Autodesk Fusion 360 part; units mm, degrees
(part 12 of 25)
  arc A2406 (61.3719, 8.262) -> (61.2504, 7.9686) centre (61.3112, 8.1153) ccw
  arc A2407 (57.5323, 7.7343) -> (57.3078, 7.9588) centre (57.4201, 7.8465) ccw
  arc A2408 (58.1296, 7.9686) -> (58.0081, 8.262) centre (58.0689, 8.1153) ccw
  arc A2409 (54.9923, 7.7343) -> (54.7678, 7.9588) centre (54.8801, 7.8465) ccw
  arc A2410 (65.6889, 8.274) -> (65.6889, 7.9565) centre (65.6889, 8.1152) ccw
  line L833 (52.07, 7.5765) -> (51.8, 7.8465)
  line L834 (58.0689, 8.1153) -> (57.42, 7.8465)
  arc A2411 (56.9749, 34.0406) -> (57.2924, 34.0406) centre (57.1337, 34.0406) ccw
  arc A2412 (56.987, 34.4786) -> (57.2804, 34.6001) centre (57.1337, 34.5394) ccw
  arc A2413 (47.9089, 8.274) -> (47.9089, 7.9565) centre (47.9089, 8.1152) ccw
  line L835 (46.72, 7.8465) -> (46.6979, 7.8557)
  arc A2414 (55.2821, 35.2406) -> (55.0576, 35.4651) centre (55.1698, 35.3528) ccw
  line L836 (46.6979, 13.1749) -> (46.7828, 13.2598)
  line L837 (53.6911, 8.1153) -> (52.9889, 8.1153)
  arc A2415 (61.3111, 7.9565) -> (61.3111, 8.274) centre (61.3111, 8.1152) ccw
  line L838 (49.8, 7.8465) -> (49.53, 7.5765)
  arc A2416 (47.3723, 7.7343) -> (47.1478, 7.9588) centre (47.2601, 7.8465) ccw
  arc A2417 (46.8951, 13.1476) -> (46.6706, 13.3721) centre (46.7829, 13.2599) ccw
  arc A2418 (46.8566, 13.1749) -> (46.5391, 13.1749) centre (46.6979, 13.1749) ccw
  arc A2419 (46.5856, 13.2872) -> (46.8102, 13.0626) centre (46.6979, 13.1749) ccw
  arc A2420 (51.1511, 7.9565) -> (51.1511, 8.274) centre (51.1511, 8.1152) ccw
  line L839 (47.26, 7.8465) -> (46.99, 7.5765)
  arc A2421 (47.1993, 7.9932) -> (47.3208, 7.6999) centre (47.2601, 7.8466) ccw
  arc A2422 (48.6719, 8.262) -> (48.5504, 7.9686) centre (48.6112, 8.1153) ccw
  arc A2423 (49.1992, 7.6999) -> (49.3207, 7.9932) centre (49.26, 7.8466) ccw
  line L840 (49.26, 7.8465) -> (48.6111, 8.1153)
  line L841 (49.53, 7.5765) -> (49.26, 7.8465)
  line L842 (46.6979, 7.8557) -> (46.6979, 13.1749)
  line L843 (46.99, 7.5765) -> (46.72, 7.8465)
  line L844 (50.4489, 8.1153) -> (49.8, 7.8465)
  line L845 (48.6111, 8.1153) -> (47.9089, 8.1153)
  line L846 (57.1337, 34.0406) -> (57.1337, 34.5394)
  line L847 (56.88, 7.8465) -> (56.2311, 8.1153)
  arc A2424 (48.6111, 7.9565) -> (48.6111, 8.274) centre (48.6111, 8.1152) ccw
  arc A2425 (46.8322, 7.9588) -> (46.6077, 7.7343) centre (46.72, 7.8465) ccw
  line L848 (54.6263, 34.5394) -> (54.6263, 34.0406)
  arc A2426 (54.2792, 7.6999) -> (54.4007, 7.9932) centre (54.34, 7.8466) ccw
  arc A2427 (49.4177, 7.6888) -> (49.6423, 7.4643) centre (49.53, 7.5765) ccw
  arc A2428 (60.6696, 7.9686) -> (60.5481, 8.262) centre (60.6089, 8.1153) ccw
  arc A2429 (53.6911, 7.9565) -> (53.6911, 8.274) centre (53.6911, 8.1152) ccw
  arc A2430 (47.9696, 7.9686) -> (47.8481, 8.262) centre (47.9089, 8.1153) ccw
  arc A2431 (54.4796, 34.6001) -> (54.773, 34.4786) centre (54.6263, 34.5393) ccw
  arc A2432 (57.0895, 35.0609) -> (56.7962, 34.9394) centre (56.9429, 35.0001) ccw
  arc A2433 (54.785, 34.5394) -> (54.4676, 34.5394) centre (54.6263, 34.5394) ccw
  line L849 (59.69, 7.5765) -> (59.42, 7.8465)
  arc A2434 (54.4676, 34.0406) -> (54.785, 34.0406) centre (54.6263, 34.0406) ccw
  line L850 (54.8172, 35.0002) -> (54.6263, 34.5394)
  arc A2435 (49.4177, 7.4643) -> (49.6423, 7.6888) centre (49.53, 7.5765) ccw
  arc A2436 (46.8777, 7.6888) -> (47.1023, 7.4643) centre (46.99, 7.5766) ccw
  arc A2437 (54.9638, 34.9394) -> (54.6705, 35.0609) centre (54.8172, 35.0002) ccw
  arc A2438 (46.6592, 7.6999) -> (46.7807, 7.9932) centre (46.7199, 7.8465) ccw
  arc A2439 (50.5096, 7.9686) -> (50.3881, 8.262) centre (50.4489, 8.1153) ccw
  line L851 (61.3111, 8.1153) -> (60.6089, 8.1153)
  line L852 (55.1698, 35.3528) -> (54.8172, 35.0002)
  line L853 (47.9089, 8.1153) -> (47.26, 7.8465)
  arc A2440 (54.4977, 7.4643) -> (54.7223, 7.6888) centre (54.61, 7.5766) ccw
  arc A2441 (53.7519, 8.262) -> (53.6304, 7.9686) centre (53.6912, 8.1153) ccw
  line L854 (57.42, 7.8465) -> (57.15, 7.5765)
  arc A2442 (54.4522, 7.9588) -> (54.2277, 7.7343) centre (54.3399, 7.8466) ccw
  arc A2443 (57.2924, 34.5394) -> (56.9749, 34.5394) centre (57.1337, 34.5394) ccw
  line L855 (56.9428, 35.0002) -> (56.5902, 35.3528)
  line L856 (54.34, 7.8465) -> (53.6911, 8.1153)
  arc A2444 (49.9123, 7.7343) -> (49.6878, 7.9588) centre (49.8, 7.8466) ccw
  arc A2445 (55.6914, 35.397) -> (55.5699, 35.6904) centre (55.6307, 35.5437) ccw
  arc A2446 (49.7393, 7.9932) -> (49.8608, 7.6999) centre (49.8, 7.8466) ccw
  arc A2447 (55.1091, 35.4995) -> (55.2306, 35.2062) centre (55.1698, 35.3529) ccw
  arc A2448 (56.5294, 35.2062) -> (56.6509, 35.4995) centre (56.5902, 35.3529) ccw
  arc A2449 (54.7049, 35.1124) -> (54.9294, 34.8879) centre (54.8172, 35.0002) ccw
  line L857 (68.0202, 17.5728) -> (67.5594, 17.7637)
  arc A2450 (56.8306, 34.8879) -> (57.0551, 35.1124) centre (56.9429, 35.0001) ccw
  arc A2451 (68.7224, 16.7594) -> (68.4049, 16.7594) centre (68.5636, 16.7594) ccw
  arc A2452 (54.9043, 18.4353) -> (55.1976, 18.5568) centre (55.051, 18.496) ccw
  arc A2453 (49.3722, 7.9588) -> (49.1477, 7.7343) centre (49.26, 7.8465) ccw
  arc A2454 (46.6362, 13.3206) -> (46.9295, 13.1991) centre (46.7828, 13.2598) ccw
  line L858 (57.1337, 34.5394) -> (56.9428, 35.0002)
  arc A2455 (56.1901, 35.6904) -> (56.0686, 35.397) centre (56.1294, 35.5437) ccw
  arc A2456 (46.8777, 7.4643) -> (47.1023, 7.6888) centre (46.99, 7.5766) ccw
  arc A2457 (55.6306, 35.7024) -> (55.6306, 35.3849) centre (55.6306, 35.5436) ccw
  line L859 (67.5594, 15.2563) -> (68.0202, 15.4472)
  arc A2458 (67.0606, 17.9224) -> (67.0606, 17.6049) centre (67.0606, 17.7636) ccw
  line L860 (67.0606, 17.7637) -> (66.5998, 17.5728)
  arc A2459 (67.5594, 17.6049) -> (67.5594, 17.9224) centre (67.5594, 17.7636) ccw
  arc A2460 (55.1632, 18.6083) -> (54.9387, 18.3838) centre (55.051, 18.496) ccw
  arc A2461 (67.9079, 15.5594) -> (68.1324, 15.3349) centre (68.0202, 15.4472) ccw
  arc A2462 (67.1214, 17.617) -> (66.9999, 17.9104) centre (67.0606, 17.7637) ccw
  arc A2463 (66.7121, 17.4606) -> (66.4876, 17.6851) centre (66.5999, 17.5728) ccw
  arc A2464 (47.1204, 13.6599) -> (46.827, 13.7814) centre (46.9737, 13.7207) ccw
  line L861 (66.5998, 15.4472) -> (67.0606, 15.2563)
  line L862 (46.7828, 13.2598) -> (46.9737, 13.7206)
  arc A2465 (66.9999, 15.1096) -> (67.1214, 15.403) centre (67.0606, 15.2563) ccw
  line L863 (67.5594, 17.7637) -> (67.0606, 17.7637)
  arc A2466 (68.2262, 15.8606) -> (68.5195, 15.7391) centre (68.3728, 15.7999) ccw
  arc A2467 (54.7898, 33.3826) -> (55.0144, 33.6072) centre (54.9021, 33.4949) ccw
  arc A2468 (68.4851, 15.6876) -> (68.2606, 15.9121) centre (68.3728, 15.7999) ccw
  arc A2469 (57.7032, 16.0683) -> (57.4787, 15.8438) centre (57.591, 15.9561) ccw
  line L864 (66.5149, 17.4879) -> (58.8251, 17.4879)
  arc A2470 (54.9294, 33.6921) -> (54.7049, 33.4676) centre (54.8172, 33.5799) ccw
  line L865 (54.9021, 33.4949) -> (54.9021, 18.8555)
  arc A2471 (46.7586, 8.0024) -> (46.6372, 7.709) centre (46.6979, 7.8557) ccw
  arc A2472 (67.9594, 17.4262) -> (68.0809, 17.7195) centre (68.0202, 17.5728) ccw
  arc A2473 (67.6201, 17.9104) -> (67.4986, 17.617) centre (67.5593, 17.7637) ccw
  line L866 (54.9021, 18.8555) -> (55.051, 18.4961)
  line L867 (55.6306, 35.5437) -> (55.1698, 35.3528)
  line L868 (66.5998, 17.5728) -> (66.5149, 17.4879)
  arc A2474 (57.9268, 15.8276) -> (57.8053, 15.5343) centre (57.8661, 15.6809) ccw
  line L869 (66.5149, 15.5321) -> (66.5998, 15.4472)
  line L870 (56.5902, 35.3528) -> (56.1294, 35.5437)
  line L871 (68.5637, 16.2606) -> (68.5637, 16.7594)
  arc A2475 (54.773, 34.1014) -> (54.4796, 33.9799) centre (54.6263, 34.0406) ccw
  arc A2476 (67.4986, 15.403) -> (67.6201, 15.1096) centre (67.5593, 15.2563) ccw
  arc A2477 (46.5391, 7.8557) -> (46.8566, 7.8557) centre (46.6979, 7.8557) ccw
  arc A2478 (66.5391, 17.7195) -> (66.6606, 17.4262) centre (66.5999, 17.5729) ccw
  line L872 (54.6263, 34.0406) -> (54.8172, 33.5798)
  arc A2479 (68.5195, 17.2809) -> (68.2262, 17.1594) centre (68.3728, 17.2202) ccw
  arc A2480 (68.1324, 17.6851) -> (67.9079, 17.4606) centre (68.0202, 17.5728) ccw
  arc A2481 (54.6705, 33.5191) -> (54.9638, 33.6406) centre (54.8172, 33.5799) ccw
  arc A2482 (68.417, 16.6986) -> (68.7104, 16.8201) centre (68.5637, 16.7594) ccw
  arc A2483 (56.7024, 35.4651) -> (56.4779, 35.2406) centre (56.5902, 35.3529) ccw
  arc A2484 (68.2606, 17.1079) -> (68.4851, 17.3324) centre (68.3728, 17.2202) ccw
  arc A2485 (58.2255, 15.6909) -> (58.2255, 15.3734) centre (58.2255, 15.5321) ccw
  line L873 (56.1294, 35.5437) -> (55.6306, 35.5437)
  arc A2486 (66.4026, 17.6002) -> (66.6272, 17.3756) centre (66.5149, 17.4879) ccw
  arc A2487 (66.6272, 15.6444) -> (66.4026, 15.4198) centre (66.5149, 15.5321) ccw
  arc A2488 (56.1294, 35.3849) -> (56.1294, 35.7024) centre (56.1294, 35.5436) ccw
  line L874 (57.8661, 15.681) -> (58.2255, 15.5321)
  line L875 (68.3728, 17.2202) -> (68.0202, 17.5728)
  arc A2489 (68.5588, 2.0638) -> (68.5588, 1.7463) centre (68.5588, 1.9051) ccw
  arc A2490 (3.696, 3.0163) -> (3.696, 3.3338) centre (3.696, 3.1751) ccw
  arc A2491 (32.964, 1.7463) -> (32.964, 2.0638) centre (32.964, 1.9051) ccw
  line L876 (55.051, 18.4961) -> (57.591, 15.9561)
  arc A2492 (5.0673, 2.6987) -> (5.0673, 2.3813) centre (5.0673, 2.54) ccw
  arc A2493 (66.6606, 15.5938) -> (66.5391, 15.3005) centre (66.5999, 15.4472) ccw
  arc A2494 (57.4787, 15.8438) -> (57.7032, 16.0683) centre (57.591, 15.9561) ccw
  line L877 (68.5637, 16.7594) -> (68.3728, 17.2202)
  arc A2495 (57.7538, 15.5687) -> (57.9783, 15.7932) centre (57.8661, 15.681) ccw
  arc A2496 (73.5277, 1.1113) -> (73.5277, 1.4287) centre (73.5277, 1.27) ccw
  arc A2497 (54.7434, 18.8555) -> (55.0609, 18.8555) centre (54.9021, 18.8555) ccw
  arc A2498 (55.0488, 18.9162) -> (54.7554, 18.7947) centre (54.9021, 18.8555) ccw
  arc A2499 (68.7104, 16.1999) -> (68.417, 16.3214) centre (68.5637, 16.2607) ccw
  arc A2500 (72.4814, 2.3813) -> (72.4814, 2.6987) centre (72.4814, 2.54) ccw
  line L878 (54.8172, 33.5798) -> (54.9021, 33.4949)
  line L879 (58.2255, 15.5321) -> (66.5149, 15.5321)
  arc A2501 (66.5149, 15.3734) -> (66.5149, 15.6909) centre (66.5149, 15.5321) ccw
  arc A2502 (58.8251, 17.6466) -> (58.8251, 17.3291) centre (58.8251, 17.4879) ccw
  arc A2503 (67.5594, 15.0976) -> (67.5594, 15.4151) centre (67.5594, 15.2564) ccw
  line L880 (56.8579, 19.4551) -> (56.8579, 33.4949)
  arc A2504 (5.0673, 2.3813) -> (5.0673, 2.6987) centre (5.0673, 2.54) ccw
  arc A2505 (68.5588, 2.6987) -> (68.5588, 2.3813) centre (68.5588, 2.54) ccw
  arc A2506 (4.331, 2.3813) -> (4.331, 2.6987) centre (4.331, 2.54) ccw
  arc A2507 (6.4386, 3.3338) -> (6.4386, 3.0163) centre (6.4386, 3.1751) ccw
  line L881 (67.0606, 15.2563) -> (67.5594, 15.2563)
  arc A2508 (67.0606, 15.4151) -> (67.0606, 15.0976) centre (67.0606, 15.2564) ccw
  arc A2509 (68.0809, 15.3005) -> (67.9594, 15.5938) centre (68.0202, 15.4472) ccw
  arc A2510 (84.2253, 2.3813) -> (84.2253, 2.6987) centre (84.2253, 2.54) ccw
  arc A2511 (66.4876, 15.3349) -> (66.7121, 15.5594) centre (66.5999, 15.4472) ccw
  arc A2512 (82.5144, 2.6987) -> (82.5144, 2.3813) centre (82.5144, 2.54) ccw
  arc A2513 (0.7747, 3.3338) -> (0.7747, 3.0163) centre (0.7747, 3.1751) ccw
  arc A2514 (58.1647, 15.3854) -> (58.2862, 15.6788) centre (58.2255, 15.5321) ccw
  arc A2515 (55.0609, 33.4949) -> (54.7434, 33.4949) centre (54.9021, 33.4949) ccw
  arc A2516 (12.6114, 3.0163) -> (12.6114, 3.3338) centre (12.6114, 3.1751) ccw
  arc A2517 (13.97, 3.3338) -> (13.97, 3.0163) centre (13.97, 3.1751) ccw
  arc A2518 (56.7456, 33.6072) -> (56.9702, 33.3826) centre (56.8579, 33.4949) ccw
  arc A2519 (68.4049, 16.2606) -> (68.7224, 16.2606) centre (68.5636, 16.2606) ccw
  arc A2520 (56.6991, 19.4551) -> (57.0166, 19.4551) centre (56.8578, 19.4551) ccw
  line L882 (56.9428, 33.5798) -> (57.1337, 34.0406)
  arc A2521 (57.2804, 33.9799) -> (56.987, 34.1014) centre (57.1337, 34.0406) ccw
  arc A2522 (5.0673, 3.3338) -> (5.0673, 3.0163) centre (5.0673, 3.1751) ccw
  arc A2523 (13.97, 3.0163) -> (13.97, 3.3338) centre (13.97, 3.1751) ccw
  line L883 (57.591, 15.9561) -> (57.8661, 15.681)
  arc A2524 (57.0551, 33.4676) -> (56.8306, 33.6921) centre (56.9429, 33.5799) ccw
  line L884 (68.0202, 15.4472) -> (68.3728, 15.7998)
  line L885 (68.3728, 15.7998) -> (68.5637, 16.2606)
  arc A2525 (5.0673, 3.0163) -> (5.0673, 3.3338) centre (5.0673, 3.1751) ccw
  arc A2526 (74.9658, 1.4287) -> (74.9658, 1.1113) centre (74.9658, 1.27) ccw
  arc A2527 (58.7128, 17.3756) -> (58.9373, 17.6002) centre (58.8251, 17.4879) ccw
  line L886 (56.8579, 33.4949) -> (56.9428, 33.5798)
  arc A2528 (40.64, 4.9212) -> (40.64, 5.2388) centre (40.64, 5.08) ccw
  arc A2529 (84.2253, 1.1113) -> (84.2253, 1.4287) centre (84.2253, 1.27) ccw
  arc A2530 (6.4132, 4.6038) -> (6.4132, 4.2862) centre (6.4132, 4.445) ccw
  arc A2531 (81.4682, 1.4287) -> (81.4682, 1.1113) centre (81.4682, 1.27) ccw
  arc A2532 (14.6936, 2.6987) -> (14.6936, 2.3813) centre (14.6936, 2.54) ccw
  arc A2533 (0.7747, 1.4287) -> (0.7747, 1.1113) centre (0.7747, 1.27) ccw
  arc A2534 (0.7747, 2.6987) -> (0.7747, 2.3813) centre (0.7747, 2.54) ccw
  arc A2535 (0.7747, 2.0638) -> (0.7747, 1.7463) centre (0.7747, 1.9051) ccw
  line L887 (58.8251, 17.4879) -> (56.8579, 19.4551)
  arc A2536 (68.5588, 1.4287) -> (68.5588, 1.1113) centre (68.5588, 1.27) ccw
  arc A2537 (33.1022, 3.6513) -> (33.1022, 3.9688) centre (33.1022, 3.81) ccw
  arc A2538 (13.97, 3.9688) -> (13.97, 3.6513) centre (13.97, 3.81) ccw
  arc A2539 (13.2464, 2.3813) -> (13.2464, 2.6987) centre (13.2464, 2.54) ccw
  arc A2540 (82.2548, 2.0638) -> (82.2548, 1.7463) centre (82.2548, 1.9051) ccw
  arc A2541 (41.4632, 5.2388) -> (41.4632, 4.9212) centre (41.4632, 5.08) ccw
  arc A2542 (15.3286, 3.3338) -> (15.3286, 3.0163) centre (15.3286, 3.1751) ccw
  arc A2543 (72.4814, 3.0163) -> (72.4814, 3.3338) centre (72.4814, 3.1751) ccw
  arc A2544 (66.5149, 17.3291) -> (66.5149, 17.6466) centre (66.5149, 17.4879) ccw
  arc A2545 (72.72, 3.6513) -> (72.72, 3.9688) centre (72.72, 3.81) ccw
  arc A2546 (13.97, 2.3813) -> (13.97, 2.6987) centre (13.97, 2.54) ccw
  arc A2547 (73.405, 4.2862) -> (73.405, 4.6038) centre (73.405, 4.445) ccw
  arc A2548 (40.64, 5.2388) -> (40.64, 4.9212) centre (40.64, 5.08) ccw
  arc A2549 (38.1, 5.2388) -> (38.1, 4.9212) centre (38.1, 5.08) ccw
  arc A2550 (41.9535, 4.9212) -> (41.9535, 5.2388) centre (41.9535, 5.08) ccw
  arc A2551 (3.9718, 4.9212) -> (3.9718, 5.2388) centre (3.9718, 5.08) ccw
  arc A2552 (34.3335, 4.9212) -> (34.3335, 5.2388) centre (34.3335, 5.08) ccw
  arc A2553 (31.7935, 4.9212) -> (31.7935, 5.2388) centre (31.7935, 5.08) ccw
  arc A2554 (39.8168, 4.9212) -> (39.8168, 5.2388) centre (39.8168, 5.08) ccw
  arc A2555 (82.5144, 3.3338) -> (82.5144, 3.0163) centre (82.5144, 3.1751) ccw
  line L888 (34.2465, 5.08) -> (34.3335, 5.08)
  line L889 (41.4632, 5.08) -> (41.9535, 5.08)
  arc A2556 (84.2253, 1.7463) -> (84.2253, 2.0638) centre (84.2253, 1.9051) ccw
  arc A2557 (5.8036, 2.6987) -> (5.8036, 2.3813) centre (5.8036, 2.54) ccw
  arc A2558 (15.0528, 5.2388) -> (15.0528, 4.9212) centre (15.0528, 5.08) ccw
  arc A2559 (80.0301, 1.1113) -> (80.0301, 1.4287) centre (80.0301, 1.27) ccw
  arc A2560 (13.97, 3.6513) -> (13.97, 3.9688) centre (13.97, 3.81) ccw
  arc A2561 (84.2253, 3.6513) -> (84.2253, 3.9688) centre (84.2253, 3.81) ccw
  arc A2562 (6.477, 3.9688) -> (6.477, 3.6513) centre (6.477, 3.81) ccw
  arc A2563 (12.8872, 4.9212) -> (12.8872, 5.2388) centre (12.8872, 5.08) ccw
  arc A2564 (13.97, 2.6987) -> (13.97, 2.3813) centre (13.97, 2.54) ccw
  arc A2565 (37.2768, 4.9212) -> (37.2768, 5.2388) centre (37.2768, 5.08) ccw
  arc A2566 (72.7411, 1.7463) -> (72.7411, 2.0638) centre (72.7411, 1.9051) ccw
  arc A2567 (32.964, 1.1113) -> (32.964, 1.4287) centre (32.964, 1.27) ccw
  arc A2568 (68.4207, 3.9688) -> (68.4207, 3.6513) centre (68.4207, 3.81) ccw
  arc A2569 (57.0166, 33.4949) -> (56.6991, 33.4949) centre (56.8578, 33.4949) ccw
  arc A2570 (84.2253, 3.0163) -> (84.2253, 3.3338) centre (84.2253, 3.1751) ccw
  arc A2571 (56.9702, 19.5673) -> (56.7456, 19.3428) centre (56.8579, 19.455) ccw
  arc A2572 (32.964, 2.3813) -> (32.964, 2.6987) centre (32.964, 2.54) ccw
  arc A2573 (56.7962, 33.6406) -> (57.0895, 33.5191) centre (56.9428, 33.5799) ccw
  arc A2574 (40.64, 5.8738) -> (40.64, 5.5562) centre (40.64, 5.715) ccw
  arc A2575 (62.1865, 5.2388) -> (62.1865, 4.9212) centre (62.1865, 5.08) ccw
  line L890 (54.5665, 5.08) -> (54.6535, 5.08)
  arc A2576 (3.4036, 6.1913) -> (3.4036, 6.5088) centre (3.4036, 6.3501) ccw
  arc A2577 (0.7747, 4.6038) -> (0.7747, 4.2862) centre (0.7747, 4.445) ccw
  arc A2578 (6.731, 6.5088) -> (6.731, 6.1913) centre (6.731, 6.3501) ccw
  arc A2579 (68.5588, 3.3338) -> (68.5588, 3.0163) centre (68.5588, 3.1751) ccw
  arc A2580 (82.2759, 3.9688) -> (82.2759, 3.6513) centre (82.2759, 3.81) ccw
  arc A2581 (52.0265, 5.2388) -> (52.0265, 4.9212) centre (52.0265, 5.08) ccw
  arc A2582 (38.9232, 5.2388) -> (38.9232, 4.9212) centre (38.9232, 5.08) ccw
  arc A2583 (62.2735, 4.9212) -> (62.2735, 5.2388) centre (62.2735, 5.08) ccw
  line L891 (59.6465, 5.08) -> (59.7335, 5.08)
  line L892 (46.9465, 5.08) -> (47.0335, 5.08)
  arc A2584 (84.2253, 4.9212) -> (84.2253, 5.2388) centre (84.2253, 5.08) ccw
  arc A2585 (36.7865, 5.2388) -> (36.7865, 4.9212) centre (36.7865, 5.08) ccw
  line L893 (38.9232, 5.08) -> (39.8168, 5.08)
  line L894 (64.7265, 5.08) -> (64.8135, 5.08)
  line L895 (67.2665, 5.08) -> (67.3535, 5.08)
  arc A2586 (15.6337, 5.8738) -> (15.6337, 5.5562) centre (15.6337, 5.715) ccw
  arc A2587 (40.64, 5.5562) -> (40.64, 5.8738) centre (40.64, 5.715) ccw
  arc A2588 (74.7818, 5.8738) -> (74.7818, 5.5562) centre (74.7818, 5.715) ccw
  arc A2589 (3.4036, 5.5562) -> (3.4036, 5.8738) centre (3.4036, 5.715) ccw
  arc A2590 (67.3535, 4.9212) -> (67.3535, 5.2388) centre (67.3535, 5.08) ccw
  arc A2591 (52.1135, 4.9212) -> (52.1135, 5.2388) centre (52.1135, 5.08) ccw
  arc A2592 (54.6535, 4.9212) -> (54.6535, 5.2388) centre (54.6535, 5.08) ccw
  arc A2593 (12.6114, 4.2862) -> (12.6114, 4.6038) centre (12.6114, 4.445) ccw
  arc A2594 (15.3286, 4.6038) -> (15.3286, 4.2862) centre (15.3286, 4.445) ccw
  arc A2595 (38.1, 4.9212) -> (38.1, 5.2388) centre (38.1, 5.08) ccw
  arc A2596 (64.7265, 5.2388) -> (64.7265, 4.9212) centre (64.7265, 5.08) ccw
  arc A2597 (32.964, 3.0163) -> (32.964, 3.3338) centre (32.964, 3.1751) ccw
  arc A2598 (0.7747, 5.2388) -> (0.7747, 4.9212) centre (0.7747, 5.08) ccw
  arc A2599 (79.9074, 4.2862) -> (79.9074, 4.6038) centre (79.9074, 4.445) ccw
  arc A2600 (44.4065, 5.2388) -> (44.4065, 4.9212) centre (44.4065, 5.08) ccw
  arc A2601 (57.1065, 5.2388) -> (57.1065, 4.9212) centre (57.1065, 5.08) ccw
  arc A2602 (12.3063, 5.5562) -> (12.3063, 5.8738) centre (12.3063, 5.715) ccw
  arc A2603 (3.7214, 4.2862) -> (3.7214, 4.6038) centre (3.7214, 4.445) ccw
  arc A2604 (64.8135, 4.9212) -> (64.8135, 5.2388) centre (64.8135, 5.08) ccw
  arc A2605 (84.2253, 5.5562) -> (84.2253, 5.8738) centre (84.2253, 5.715) ccw
  arc A2606 (34.2465, 5.2388) -> (34.2465, 4.9212) centre (34.2465, 5.08) ccw
  arc A2607 (44.4935, 4.9212) -> (44.4935, 5.2388) centre (44.4935, 5.08) ccw
  line L896 (36.7865, 5.08) -> (37.2768, 5.08)
  arc A2608 (73.7116, 5.5562) -> (73.7116, 5.8738) centre (73.7116, 5.715) ccw
  arc A2609 (84.2253, 4.2862) -> (84.2253, 4.6038) centre (84.2253, 4.445) ccw
  arc A2610 (0.7747, 3.9688) -> (0.7747, 3.6513) centre (0.7747, 3.81) ccw
  arc A2611 (3.6576, 3.6513) -> (3.6576, 3.9688) centre (3.6576, 3.81) ccw
  arc A2612 (49.4865, 5.2388) -> (49.4865, 4.9212) centre (49.4865, 5.08) ccw
  arc A2613 (75.0884, 4.6038) -> (75.0884, 4.2862) centre (75.0884, 4.445) ccw
  arc A2614 (59.7335, 4.9212) -> (59.7335, 5.2388) centre (59.7335, 5.08) ccw
  arc A2615 (69.8065, 5.2388) -> (69.8065, 4.9212) centre (69.8065, 5.08) ccw
  arc A2616 (6.1628, 5.2388) -> (6.1628, 4.9212) centre (6.1628, 5.08) ccw
  arc A2617 (81.5908, 4.6038) -> (81.5908, 4.2862) centre (81.5908, 4.445) ccw
  arc A2618 (29.4986, 5.5562) -> (29.4986, 5.8738) centre (29.4986, 5.715) ccw
  arc A2619 (38.1, 5.8738) -> (38.1, 5.5562) centre (38.1, 5.715) ccw
  arc A2620 (44.4935, 7.4612) -> (44.4935, 7.7788) centre (44.4935, 7.62) ccw
  arc A2621 (40.64, 6.8262) -> (40.64, 7.1438) centre (40.64, 6.985) ccw
  arc A2622 (82.1916, 6.5088) -> (82.1916, 6.1913) centre (82.1916, 6.3501) ccw
  arc A2623 (57.1935, 4.9212) -> (57.1935, 5.2388) centre (57.1935, 5.08) ccw
  arc A2624 (80.214, 5.5562) -> (80.214, 5.8738) centre (80.214, 5.715) ccw
  arc A2625 (31.7935, 7.4612) -> (31.7935, 7.7788) centre (31.7935, 7.62) ccw
  arc A2626 (34.2465, 7.7788) -> (34.2465, 7.4612) centre (34.2465, 7.62) ccw
  arc A2627 (46.9465, 5.2388) -> (46.9465, 4.9212) centre (46.9465, 5.08) ccw
  arc A2628 (41.4632, 7.7788) -> (41.4632, 7.4612) centre (41.4632, 7.62) ccw
  arc A2629 (54.5665, 5.2388) -> (54.5665, 4.9212) centre (54.5665, 5.08) ccw
  arc A2630 (3.9972, 7.4612) -> (3.9972, 7.7788) centre (3.9972, 7.62) ccw
  arc A2631 (40.64, 7.1438) -> (40.64, 6.8262) centre (40.64, 6.985) ccw
  arc A2632 (12.3063, 6.1913) -> (12.3063, 6.5088) centre (12.3063, 6.3501) ccw
  arc A2633 (15.6337, 6.5088) -> (15.6337, 6.1913) centre (15.6337, 6.3501) ccw
  arc A2634 (49.5735, 4.9212) -> (49.5735, 5.2388) centre (49.5735, 5.08) ccw
  arc A2635 (70.7429, 6.8262) -> (70.7429, 7.1438) centre (70.7429, 6.985) ccw
  arc A2636 (0.7747, 7.7788) -> (0.7747, 7.4612) centre (0.7747, 7.62) ccw
  line L897 (57.1065, 5.08) -> (57.1935, 5.08)
  line L898 (62.1865, 5.08) -> (62.2735, 5.08)
  arc A2637 (0.7747, 6.5088) -> (0.7747, 6.1913) centre (0.7747, 6.3501) ccw
  arc A2638 (67.2665, 5.2388) -> (67.2665, 4.9212) centre (67.2665, 5.08) ccw
  arc A2639 (38.1, 7.7788) -> (38.1, 7.4612) centre (38.1, 7.62) ccw
  arc A2640 (70.2277, 7.1438) -> (70.2277, 6.8262) centre (70.2277, 6.985) ccw
  arc A2641 (34.3335, 7.4612) -> (34.3335, 7.7788) centre (34.3335, 7.62) ccw
  arc A2642 (79.3067, 6.1913) -> (79.3067, 6.5088) centre (79.3067, 6.3501) ccw
  line L899 (38.1, 6.35) -> (40.64, 6.35)
  arc A2643 (15.6337, 7.1438) -> (15.6337, 6.8262) centre (15.6337, 6.985) ccw
  arc A2644 (38.1, 5.5562) -> (38.1, 5.8738) centre (38.1, 5.715) ccw
  arc A2645 (0.7747, 5.8738) -> (0.7747, 5.5562) centre (0.7747, 5.715) ccw
  arc A2646 (59.6465, 5.2388) -> (59.6465, 4.9212) centre (59.6465, 5.08) ccw
  arc A2647 (75.6891, 6.5088) -> (75.6891, 6.1913) centre (75.6891, 6.3501) ccw
  arc A2648 (40.64, 7.7788) -> (40.64, 7.4612) centre (40.64, 7.62) ccw
  arc A2649 (6.731, 5.8738) -> (6.731, 5.5562) centre (6.731, 5.715) ccw
  line L900 (46.9465, 7.62) -> (47.0335, 7.62)
  arc A2650 (40.64, 6.1913) -> (40.64, 6.5088) centre (40.64, 6.3501) ccw
  arc A2651 (47.0335, 7.4612) -> (47.0335, 7.7788) centre (47.0335, 7.62) ccw
  arc A2652 (6.1374, 7.7788) -> (6.1374, 7.4612) centre (6.1374, 7.62) ccw
  arc A2653 (3.4036, 6.8262) -> (3.4036, 7.1438) centre (3.4036, 6.985) ccw
  arc A2654 (38.1, 6.8262) -> (38.1, 7.1438) centre (38.1, 6.985) ccw
  arc A2655 (0.7747, 7.1438) -> (0.7747, 6.8262) centre (0.7747, 6.985) ccw
  arc A2656 (11.317, 7.4612) -> (11.317, 7.7788) centre (11.317, 7.62) ccw
  arc A2657 (81.2842, 5.8738) -> (81.2842, 5.5562) centre (81.2842, 5.715) ccw
  arc A2658 (28.8636, 6.1913) -> (28.8636, 6.5088) centre (28.8636, 6.3501) ccw
  arc A2659 (70.2277, 5.8738) -> (70.2277, 5.5562) centre (70.2277, 5.715) ccw
  line L901 (44.4065, 5.08) -> (44.4935, 5.08)
  arc A2660 (38.1, 7.1438) -> (38.1, 6.8262) centre (38.1, 6.985) ccw
  arc A2661 (41.9535, 7.4612) -> (41.9535, 7.7788) centre (41.9535, 7.62) ccw
  line L902 (49.4865, 5.08) -> (49.5735, 5.08)
  arc A2662 (47.0335, 4.9212) -> (47.0335, 5.2388) centre (47.0335, 5.08) ccw
  line L903 (52.0265, 5.08) -> (52.1135, 5.08)
  arc A2663 (11.952, 6.8262) -> (11.952, 7.1438) centre (11.952, 6.985) ccw
  arc A2664 (59.6465, 7.7788) -> (59.6465, 7.4612) centre (59.6465, 7.62) ccw
  arc A2665 (84.2253, 8.0963) -> (84.2253, 8.4138) centre (84.2253, 8.2551) ccw
  arc A2666 (54.6535, 7.4612) -> (54.6535, 7.7788) centre (54.6535, 7.62) ccw
  arc A2667 (40.64, 7.4612) -> (40.64, 7.7788) centre (40.64, 7.62) ccw
  line L904 (49.4865, 7.62) -> (49.5735, 7.62)
  line L905 (62.1865, 7.62) -> (62.2735, 7.62)
  arc A2668 (26.3236, 8.7313) -> (26.3236, 9.0488) centre (26.3236, 8.89) ccw
  arc A2669 (82.983, 8.4138) -> (82.983, 8.0963) centre (82.983, 8.2551) ccw
  arc A2670 (37.2768, 7.4612) -> (37.2768, 7.7788) centre (37.2768, 7.62) ccw
  line L906 (34.2465, 7.62) -> (34.3335, 7.62)
  arc A2671 (44.4065, 7.7788) -> (44.4065, 7.4612) centre (44.4065, 7.62) ccw
  arc A2672 (30.8264, 7.7788) -> (30.8264, 7.4612) centre (30.8264, 7.62) ccw
  arc A2673 (84.2253, 6.8262) -> (84.2253, 7.1438) centre (84.2253, 6.985) ccw
  arc A2674 (72.8043, 6.1913) -> (72.8043, 6.5088) centre (72.8043, 6.3501) ccw
  arc A2675 (54.5665, 7.7788) -> (54.5665, 7.4612) centre (54.5665, 7.62) ccw
  arc A2676 (15.0528, 7.7788) -> (15.0528, 7.4612) centre (15.0528, 7.62) ccw
  arc A2677 (27.5936, 7.4612) -> (27.5936, 7.7788) centre (27.5936, 7.62) ccw
  arc A2678 (44.7421, 8.0963) -> (44.7421, 8.4138) centre (44.7421, 8.2551) ccw
  arc A2679 (38.1, 7.4612) -> (38.1, 7.7788) centre (38.1, 7.62) ccw
  arc A2680 (39.8168, 7.4612) -> (39.8168, 7.7788) centre (39.8168, 7.62) ccw
  arc A2681 (52.1135, 7.4612) -> (52.1135, 7.7788) centre (52.1135, 7.62) ccw
  line L907 (69.8065, 7.62) -> (70.1079, 7.62)
  arc A2682 (26.9586, 8.0963) -> (26.9586, 8.4138) centre (26.9586, 8.2551) ccw
  arc A2683 (28.2286, 6.8262) -> (28.2286, 7.1438) centre (28.2286, 6.985) ccw
  arc A2684 (84.2253, 6.1913) -> (84.2253, 6.5088) centre (84.2253, 6.3501) ccw
  arc A2685 (82.4863, 7.1438) -> (82.4863, 6.8262) centre (82.4863, 6.985) ccw
  arc A2686 (13.448, 8.4138) -> (13.448, 8.0963) centre (13.448, 8.2551) ccw
  arc A2687 (70.3453, 6.5088) -> (70.3453, 6.1913) centre (70.3453, 6.3501) ccw
  arc A2688 (46.9465, 7.7788) -> (46.9465, 7.4612) centre (46.9465, 7.62) ccw
  arc A2689 (29.5564, 9.0488) -> (29.5564, 8.7313) centre (29.5564, 8.89) ccw
  arc A2690 (46.6979, 8.4138) -> (46.6979, 8.0963) centre (46.6979, 8.2551) ccw
  arc A2691 (38.1, 6.5088) -> (38.1, 6.1913) centre (38.1, 6.3501) ccw
  arc A2692 (52.0265, 7.7788) -> (52.0265, 7.4612) centre (52.0265, 7.62) ccw
  line L908 (57.1065, 7.62) -> (57.1935, 7.62)
  arc A2693 (59.7335, 7.4612) -> (59.7335, 7.7788) centre (59.7335, 7.62) ccw
  line L909 (64.7265, 7.62) -> (64.8135, 7.62)
  arc A2694 (38.9232, 7.7788) -> (38.9232, 7.4612) centre (38.9232, 7.62) ccw
  arc A2695 (67.2665, 7.7788) -> (67.2665, 7.4612) centre (67.2665, 7.62) ccw
  arc A2696 (69.4729, 8.0963) -> (69.4729, 8.4138) centre (69.4729, 8.2551) ccw
  arc A2697 (36.7865, 7.7788) -> (36.7865, 7.4612) centre (36.7865, 7.62) ccw
  arc A2698 (46.6979, 9.0488) -> (46.6979, 8.7313) centre (46.6979, 8.89) ccw
  arc A2699 (6.731, 7.1438) -> (6.731, 6.8262) centre (6.731, 6.985) ccw
  arc A2700 (68.8379, 8.7313) -> (68.8379, 9.0488) centre (68.8379, 8.89) ccw
  arc A2701 (82.5144, 7.7788) -> (82.5144, 7.4612) centre (82.5144, 7.62) ccw
  arc A2702 (64.8135, 7.4612) -> (64.8135, 7.7788) centre (64.8135, 7.62) ccw
  line L910 (59.6465, 7.62) -> (59.7335, 7.62)
  arc A2703 (4.1275, 8.7313) -> (4.1275, 9.0488) centre (4.1275, 8.89) ccw
  line L911 (52.0265, 7.62) -> (52.1135, 7.62)
  arc A2704 (84.2253, 8.7313) -> (84.2253, 9.0488) centre (84.2253, 8.89) ccw
  arc A2705 (0.7747, 10.3187) -> (0.7747, 10.0013) centre (0.7747, 10.16) ccw
  arc A2706 (30.1914, 8.4138) -> (30.1914, 8.0963) centre (30.1914, 8.2551) ccw
  arc A2707 (28.2864, 10.3187) -> (28.2864, 10.0013) centre (28.2864, 10.16) ccw
  arc A2708 (10.4521, 8.7313) -> (10.4521, 9.0488) centre (10.4521, 8.89) ccw
  arc A2709 (67.3535, 7.4612) -> (67.3535, 7.7788) centre (67.3535, 7.62) ccw
  line L912 (54.5665, 7.62) -> (54.6535, 7.62)
  arc A2710 (64.7265, 7.7788) -> (64.7265, 7.4612) centre (64.7265, 7.62) ccw
  arc A2711 (79.7385, 8.7313) -> (79.7385, 9.0488) centre (79.7385, 8.89) ccw
  arc A2712 (57.1065, 7.7788) -> (57.1065, 7.4612) centre (57.1065, 7.62) ccw
  arc A2713 (3.6263, 10.6363) -> (3.6263, 10.9537) centre (3.6263, 10.795) ccw
  arc A2714 (14.4213, 10.0013) -> (14.4213, 10.3187) centre (14.4213, 10.16) ccw
  arc A2715 (12.813, 9.0488) -> (12.813, 8.7313) centre (12.813, 8.89) ccw
  arc A2716 (12.4079, 10.3187) -> (12.4079, 10.0013) centre (12.4079, 10.16) ccw
  arc A2717 (81.6991, 10.0013) -> (81.6991, 10.3187) centre (81.6991, 10.16) ccw
  arc A2718 (6.0833, 9.6837) -> (6.0833, 9.3663) centre (6.0833, 9.525) ccw
  arc A2719 (84.2253, 7.4612) -> (84.2253, 7.7788) centre (84.2253, 7.62) ccw
  arc A2720 (62.1865, 7.7788) -> (62.1865, 7.4612) centre (62.1865, 7.62) ccw
  arc A2721 (69.8065, 7.7788) -> (69.8065, 7.4612) centre (69.8065, 7.62) ccw
  arc A2722 (46.6979, 10.3187) -> (46.6979, 10.0013) centre (46.6979, 10.16) ccw
  arc A2723 (66.0563, 10.0013) -> (66.0563, 10.3187) centre (66.0563, 10.16) ccw
  arc A2724 (76.313, 10.3187) -> (76.313, 10.0013) centre (76.313, 10.16) ccw
  arc A2725 (6.0833, 9.0488) -> (6.0833, 8.7313) centre (6.0833, 8.89) ccw
  arc A2726 (84.2253, 10.0013) -> (84.2253, 10.3187) centre (84.2253, 10.16) ccw
  arc A2727 (70.372, 10.0013) -> (70.372, 10.3187) centre (70.372, 10.16) ccw
  arc A2728 (83.6549, 10.3187) -> (83.6549, 10.0013) centre (83.6549, 10.16) ccw
  arc A2729 (49.4865, 7.7788) -> (49.4865, 7.4612) centre (49.4865, 7.62) ccw
  arc A2730 (4.1275, 10.0013) -> (4.1275, 10.3187) centre (4.1275, 10.16) ccw
  arc A2731 (83.5524, 9.0488) -> (83.5524, 8.7313) centre (83.5524, 8.89) ccw
  arc A2732 (6.0833, 8.4138) -> (6.0833, 8.0963) centre (6.0833, 8.2551) ccw
  arc A2733 (71.007, 9.3663) -> (71.007, 9.6837) centre (71.007, 9.525) ccw
  arc A2734 (57.1935, 7.4612) -> (57.1935, 7.7788) centre (57.1935, 7.62) ccw
  arc A2735 (0.7747, 10.9537) -> (0.7747, 10.6363) centre (0.7747, 10.795) ccw
  arc A2736 (10.682, 8.0963) -> (10.682, 8.4138) centre (10.682, 8.2551) ccw
  arc A2737 (25.0536, 10.0013) -> (25.0536, 10.3187) centre (25.0536, 10.16) ccw
  arc A2738 (28.9214, 9.6837) -> (28.9214, 9.3663) centre (28.9214, 9.525) ccw
  arc A2739 (0.7747, 8.4138) -> (0.7747, 8.0963) centre (0.7747, 8.2551) ccw
  arc A2740 (44.7421, 8.7313) -> (44.7421, 9.0488) centre (44.7421, 8.89) ccw
  line L913 (67.2665, 7.62) -> (67.3535, 7.62)
  arc A2741 (4.1275, 8.0963) -> (4.1275, 8.4138) centre (4.1275, 8.2551) ccw
  arc A2742 (16.1095, 10.3187) -> (16.1095, 10.0013) centre (16.1095, 10.16) ccw
  arc A2743 (83.6549, 9.6837) -> (83.6549, 9.3663) centre (83.6549, 9.525) ccw
  arc A2744 (62.2735, 7.4612) -> (62.2735, 7.7788) centre (62.2735, 7.62) ccw
  arc A2745 (71.6038, 9.0488) -> (71.6038, 8.7313) centre (71.6038, 8.89) ccw
  arc A2746 (70.1079, 7.4612) -> (70.1079, 7.7788) centre (70.1079, 7.62) ccw
  arc A2747 (0.7747, 9.0488) -> (0.7747, 8.7313) centre (0.7747, 8.89) ccw
  arc A2748 (49.5735, 7.4612) -> (49.5735, 7.7788) centre (49.5735, 7.62) ccw
  arc A2749 (70.3338, 10.3187) -> (70.3338, 10.0013) centre (70.3338, 10.16) ccw
  arc A2750 (25.6886, 9.3663) -> (25.6886, 9.6837) centre (25.6886, 9.525) ccw
  line L914 (70.3338, 10.16) -> (70.372, 10.16)
  line L915 (70.9688, 9.525) -> (71.007, 9.525)
  arc A2751 (12.4079, 9.6837) -> (12.4079, 9.3663) centre (12.4079, 9.525) ccw
  arc A2752 (84.2253, 9.3663) -> (84.2253, 9.6837) centre (84.2253, 9.525) ccw
  arc A2753 (81.4871, 9.3663) -> (81.4871, 9.6837) centre (81.4871, 9.525) ccw
  arc A2754 (69.102, 11.2713) -> (69.102, 11.5887) centre (69.102, 11.43) ccw
  arc A2755 (81.5916, 11.2713) -> (81.5916, 11.5887) centre (81.5916, 11.43) ccw
  arc A2756 (13.7795, 11.2713) -> (13.7795, 11.5887) centre (13.7795, 11.43) ccw
  arc A2757 (6.0833, 10.3187) -> (6.0833, 10.0013) centre (6.0833, 10.16) ccw
  arc A2758 (0.7747, 9.6837) -> (0.7747, 9.3663) centre (0.7747, 9.525) ccw
  arc A2759 (0.7747, 11.5887) -> (0.7747, 11.2713) centre (0.7747, 11.43) ccw
  arc A2760 (44.7421, 10.6363) -> (44.7421, 10.9537) centre (44.7421, 10.795) ccw
  arc A2761 (77.583, 11.5887) -> (77.583, 11.2713) centre (77.583, 11.43) ccw
  arc A2762 (66.216, 9.3663) -> (66.216, 9.6837) centre (66.216, 9.525) ccw
  arc A2763 (70.9688, 9.6837) -> (70.9688, 9.3663) centre (70.9688, 9.525) ccw
  arc A2764 (16.8945, 11.5887) -> (16.8945, 11.2713) centre (16.8945, 11.43) ccw
  arc A2765 (27.0164, 11.5887) -> (27.0164, 11.2713) centre (27.0164, 11.43) ccw
  arc A2766 (84.2253, 11.2713) -> (84.2253, 11.5887) centre (84.2253, 11.43) ccw
  arc A2767 (44.7421, 10.0013) -> (44.7421, 10.3187) centre (44.7421, 10.16) ccw
  arc A2768 (10.4521, 10.0013) -> (10.4521, 10.3187) centre (10.4521, 10.16) ccw
  arc A2769 (13.8117, 11.9063) -> (13.8117, 12.2238) centre (13.8117, 12.0651) ccw
  arc A2770 (12.178, 12.2238) -> (12.178, 11.9063) centre (12.178, 12.0651) ccw
  arc A2771 (75.678, 9.6837) -> (75.678, 9.3663) centre (75.678, 9.525) ccw
  arc A2772 (10.4521, 9.3663) -> (10.4521, 9.6837) centre (10.4521, 9.525) ccw
  arc A2773 (76.948, 10.9537) -> (76.948, 10.6363) centre (76.948, 10.795) ccw
  arc A2774 (4.1275, 9.3663) -> (4.1275, 9.6837) centre (4.1275, 9.525) ccw
  arc A2775 (24.4185, 10.6363) -> (24.4185, 10.9537) centre (24.4185, 10.795) ccw
  arc A2776 (73.2432, 11.5887) -> (73.2432, 11.2713) centre (73.2432, 11.43) ccw
  arc A2777 (10.047, 11.2713) -> (10.047, 11.5887) centre (10.047, 11.43) ccw
  arc A2778 (13.7863, 10.6363) -> (13.7863, 10.9537) centre (13.7863, 10.795) ccw
  arc A2779 (23.7836, 11.2713) -> (23.7836, 11.5887) centre (23.7836, 11.43) ccw
  arc A2780 (84.2253, 10.6363) -> (84.2253, 10.9537) centre (84.2253, 10.795) ccw
  arc A2781 (73.2361, 8.7313) -> (73.2361, 9.0488) centre (73.2361, 8.89) ccw
  arc A2782 (66.216, 10.6363) -> (66.216, 10.9537) centre (66.216, 10.795) ccw
  arc A2783 (69.737, 10.6363) -> (69.737, 10.9537) centre (69.737, 10.795) ccw
  arc A2784 (3.6195, 11.2713) -> (3.6195, 11.5887) centre (3.6195, 11.43) ccw
  line L916 (69.6988, 10.795) -> (69.737, 10.795)
  arc A2785 (46.6979, 10.9537) -> (46.6979, 10.6363) centre (46.6979, 10.795) ccw
  arc A2786 (12.4079, 10.9537) -> (12.4079, 10.6363) centre (12.4079, 10.795) ccw
  arc A2787 (75.2573, 9.0488) -> (75.2573, 8.7313) centre (75.2573, 8.89) ccw
  arc A2788 (44.7421, 9.3663) -> (44.7421, 9.6837) centre (44.7421, 9.525) ccw
  arc A2789 (46.6979, 9.6837) -> (46.6979, 9.3663) centre (46.6979, 9.525) ccw
  arc A2790 (8.777, 12.5413) -> (8.777, 12.8588) centre (8.777, 12.7001) ccw
  arc A2791 (71.6638, 13.1763) -> (71.6638, 13.4938) centre (71.6638, 13.335) ccw
  arc A2792 (26.3814, 12.2238) -> (26.3814, 11.9063) centre (26.3814, 12.0651) ccw
  arc A2793 (44.7421, 11.2713) -> (44.7421, 11.5887) centre (44.7421, 11.43) ccw
  arc A2794 (27.6514, 10.9537) -> (27.6514, 10.6363) centre (27.6514, 10.795) ccw
  arc A2795 (72.517, 12.8588) -> (72.517, 12.5413) centre (72.517, 12.7001) ccw
  arc A2796 (23.1486, 11.9063) -> (23.1486, 12.2238) centre (23.1486, 12.0651) ccw
  arc A2797 (12.4079, 11.5887) -> (12.4079, 11.2713) centre (12.4079, 11.43) ccw
  arc A2798 (69.6988, 10.9537) -> (69.6988, 10.6363) centre (69.6988, 10.795) ccw
  arc A2799 (6.5845, 10.9537) -> (6.5845, 10.6363) centre (6.5845, 10.795) ccw
  arc A2800 (0.7747, 12.2238) -> (0.7747, 11.9063) centre (0.7747, 12.0651) ccw
  arc A2801 (72.517, 11.2713) -> (72.517, 11.5887) centre (72.517, 11.43) ccw
  arc A2802 (46.6979, 11.5887) -> (46.6979, 11.2713) centre (46.6979, 11.43) ccw
  arc A2803 (46.814, 13.4938) -> (46.814, 13.1763) centre (46.814, 13.335) ccw
  arc A2804 (84.1629, 12.2238) -> (84.1629, 11.9063) centre (84.1629, 12.0651) ccw
  arc A2805 (81.6991, 10.6363) -> (81.6991, 10.9537) centre (81.6991, 10.795) ccw
  arc A2806 (84.2253, 11.9063) -> (84.2253, 12.2238) centre (84.2253, 12.0651) ccw
  arc A2807 (83.7624, 11.5887) -> (83.7624, 11.2713) centre (83.7624, 11.43) ccw
  arc A2808 (16.7445, 10.9537) -> (16.7445, 10.6363) centre (16.7445, 10.795) ccw
  arc A2809 (0.7747, 12.8588) -> (0.7747, 12.5413) centre (0.7747, 12.7001) ccw
  arc A2810 (69.963, 13.4938) -> (69.963, 13.1763) centre (69.963, 13.335) ccw
  arc A2811 (6.5913, 11.5887) -> (6.5913, 11.2713) centre (6.5913, 11.43) ccw
  arc A2812 (72.517, 12.2238) -> (72.517, 11.9063) centre (72.517, 12.0651) ccw
  arc A2813 (10.4521, 10.6363) -> (10.4521, 10.9537) centre (10.4521, 10.795) ccw
  arc A2814 (9.412, 11.9063) -> (9.412, 12.2238) centre (9.412, 12.0651) ccw
  arc A2815 (15.5667, 13.1763) -> (15.5667, 13.4938) centre (15.5667, 13.335) ccw
  arc A2816 (78.218, 12.2238) -> (78.218, 11.9063) centre (78.218, 12.0651) ccw
  arc A2817 (22.5714, 12.2238) -> (22.5714, 11.9063) centre (22.5714, 12.0651) ccw
  arc A2818 (5.9241, 12.8588) -> (5.9241, 12.5413) centre (5.9241, 12.7001) ccw
  arc A2819 (68.467, 11.9063) -> (68.467, 12.2238) centre (68.467, 12.0651) ccw
  line L917 (71.233, 12.065) -> (71.2851, 12.065)
  arc A2820 (74.817, 11.2713) -> (74.817, 11.5887) centre (74.817, 11.43) ccw
  arc A2821 (25.1114, 13.4938) -> (25.1114, 13.1763) centre (25.1114, 13.335) ccw
  arc A2822 (6.5591, 12.2238) -> (6.5591, 11.9063) centre (6.5591, 12.0651) ccw
  arc A2823 (44.7421, 12.5413) -> (44.7421, 12.8588) centre (44.7421, 12.7001) ccw
  arc A2824 (72.517, 11.5887) -> (72.517, 11.2713) centre (72.517, 11.43) ccw
  arc A2825 (84.1629, 12.8588) -> (84.1629, 12.5413) centre (84.1629, 12.7001) ccw
  arc A2826 (44.626, 13.1763) -> (44.626, 13.4938) centre (44.626, 13.335) ccw
  arc A2827 (48.782, 13.1763) -> (48.782, 13.4938) centre (48.782, 13.335) ccw
  arc A2828 (0.7747, 13.4938) -> (0.7747, 13.1763) centre (0.7747, 13.335) ccw
  arc A2829 (10.908, 13.4938) -> (10.908, 13.1763) centre (10.908, 13.335) ccw
  arc A2830 (78.853, 12.8588) -> (78.853, 12.5413) centre (78.853, 12.7001) ccw
  arc A2831 (83.6549, 10.9537) -> (83.6549, 10.6363) centre (83.6549, 10.795) ccw
  arc A2832 (73.7489, 12.8588) -> (73.7489, 12.5413) centre (73.7489, 12.7001) ccw
  arc A2833 (3.6517, 11.9063) -> (3.6517, 12.2238) centre (3.6517, 12.0651) ccw
  arc A2834 (20.4787, 38.1) -> (20.1612, 38.1) centre (20.32, 38.1) ccw
  line L918 (20.32, 36.8681) -> (20.32, 38.1)
  arc A2835 (18.9206, 36.918) -> (19.1073, 37.1748) centre (19.014, 37.0464) ccw
  line L919 (20.32, 38.1) -> (20.32, 36.8681)
  arc A2836 (18.8322, 37.4097) -> (18.6077, 37.1852) centre (18.72, 37.2975) ccw
  arc A2837 (21.8762, 37.0319) -> (21.6896, 37.2888) centre (21.7829, 37.1604) ccw
  line L920 (18.518, 37.6271) -> (18.606, 37.4543)
  arc A2838 (21.5327, 37.1748) -> (21.7194, 36.918) centre (21.6261, 37.0464) ccw
  arc A2839 (21.0525, 37.0249) -> (21.1022, 36.7113) centre (21.0773, 36.8681) ccw
  line L921 (18.606, 37.4543) -> (18.72, 37.2975)
  arc A2840 (20.32, 38.2587) -> (20.32, 37.9412) centre (20.32, 38.0999) ccw
  arc A2841 (19.086, 37.1878) -> (18.9419, 36.9049) centre (19.014, 37.0464) ccw
  line L922 (20.32, 38.1) -> (18.4277, 38.1)
  arc A2842 (21.0774, 36.7094) -> (21.0774, 37.0268) centre (21.0774, 36.8681) ccw
  arc A2843 (18.7448, 37.0481) -> (18.9693, 37.2726) centre (18.8571, 37.1603) ccw
  arc A2844 (21.6981, 36.9049) -> (21.554, 37.1878) centre (21.6261, 37.0464) ccw
  arc A2845 (18.7344, 37.5477) -> (18.4776, 37.361) centre (18.606, 37.4543) ccw
  arc A2846 (21.3812, 37.0998) -> (21.5254, 36.8169) centre (21.4533, 36.9583) ccw
  line L923 (18.458, 37.8115) -> (18.518, 37.6271)
  arc A2847 (18.3012, 37.7867) -> (18.6148, 37.8364) centre (18.458, 37.8115) ccw
  line L924 (21.0774, 36.8681) -> (21.2689, 36.8984)
  arc A2848 (19.5378, 36.7113) -> (19.5875, 37.0249) centre (19.5627, 36.8681) ccw
  arc A2849 (18.367, 37.5781) -> (18.6689, 37.6762) centre (18.5179, 37.6272) ccw
  arc A2850 (18.6594, 37.6992) -> (18.3765, 37.555) centre (18.5179, 37.6271) ccw
  arc A2851 (20.1612, 38.1) -> (20.4787, 38.1) centre (20.32, 38.1) ccw
  arc A2852 (19.5626, 37.0268) -> (19.5626, 36.7094) centre (19.5626, 36.8681) ccw
  arc A2853 (18.269, 38.003) -> (18.5865, 38.003) centre (18.4277, 38.003) ccw
  arc A2854 (18.4277, 38.2588) -> (18.4277, 37.9413) centre (18.4277, 38.1) ccw
  line L925 (21.2689, 36.8984) -> (21.4533, 36.9584)
  line L926 (19.3711, 36.8984) -> (19.5626, 36.8681)
  arc A2855 (20.1612, 36.8681) -> (20.4787, 36.8681) centre (20.32, 36.8681) ccw
  arc A2856 (19.2358, 37.1093) -> (19.1377, 36.8074) centre (19.1867, 36.9583) ccw
  arc A2857 (18.5865, 38.1) -> (18.269, 38.1) centre (18.4277, 38.1) ccw
  arc A2858 (20.4787, 38.1) -> (20.1612, 38.1) centre (20.32, 38.1) ccw
  arc A2859 (19.1146, 36.8169) -> (19.2588, 37.0998) centre (19.1867, 36.9584) ccw
  arc A2860 (21.5406, 39.3753) -> (21.3965, 39.0924) centre (21.4686, 39.2339) ccw
  arc A2861 (20.32, 37.9413) -> (20.32, 38.2588) centre (20.32, 38.1) ccw
  arc A2862 (20.32, 37.9412) -> (20.32, 38.2587) centre (20.32, 38.0999) ccw
  line L927 (18.4277, 38.1) -> (18.4277, 38.003)
  arc A2863 (18.5845, 38.0279) -> (18.2709, 37.9782) centre (18.4277, 38.0031) ccw
  line L928 (20.32, 36.8681) -> (21.0774, 36.8681)
  arc A2864 (18.4277, 38.2587) -> (18.4277, 37.9412) centre (18.4277, 38.0999) ccw
  arc A2865 (21.5023, 36.8074) -> (21.4042, 37.1093) centre (21.4533, 36.9583) ccw
  line L929 (18.4277, 38.1) -> (20.32, 38.1)
  arc A2866 (18.9504, 37.2888) -> (18.7638, 37.0319) centre (18.8571, 37.1604) ccw
  arc A2867 (19.3221, 36.7475) -> (19.4202, 37.0494) centre (19.3712, 36.8984) ccw
  arc A2868 (20.32, 36.7093) -> (20.32, 37.0268) centre (20.32, 36.8681) ccw
  line L930 (19.1867, 36.9584) -> (19.3711, 36.8984)
  line L931 (19.5626, 36.8681) -> (20.32, 36.8681)
  arc A2869 (18.5915, 37.2042) -> (18.8484, 37.3908) centre (18.72, 37.2975) ccw
  arc A2870 (20.1613, 36.8681) -> (20.4788, 36.8681) centre (20.3201, 36.8681) ccw
  arc A2871 (20.4788, 38.1) -> (20.1613, 38.1) centre (20.3201, 38.1) ccw
  arc A2872 (21.2198, 37.0494) -> (21.3179, 36.7475) centre (21.2688, 36.8984) ccw
  line L932 (21.6261, 37.0464) -> (21.7829, 37.1604)
  line L933 (18.4277, 38.003) -> (18.458, 37.8115)
  arc A2873 (20.32, 37.9412) -> (20.32, 38.2587) centre (20.32, 38.0999) ccw
  line L934 (18.72, 37.2975) -> (18.8571, 37.1604)
  arc A2874 (18.4645, 37.3823) -> (18.7474, 37.5264) centre (18.6059, 37.4544) ccw
  arc A2875 (18.609, 37.8606) -> (18.3071, 37.7625) centre (18.4581, 37.8116) ccw
  arc A2876 (19.396, 37.0552) -> (19.3463, 36.7416) centre (19.3712, 36.8984) ccw
  line L935 (19.0139, 37.0464) -> (19.1867, 36.9584)
  line L936 (18.8571, 37.1604) -> (19.0139, 37.0464)
  arc A2877 (20.32, 37.0268) -> (20.32, 36.7094) centre (20.32, 36.8681) ccw
  arc A2878 (22.0252, 37.8364) -> (22.3388, 37.7867) centre (22.182, 37.8115) ccw
  arc A2879 (20.32, 38.2588) -> (20.32, 37.9413) centre (20.32, 38.1) ccw
  arc A2880 (21.554, 39.0122) -> (21.6981, 39.2951) centre (21.6261, 39.1536) ccw
  line L937 (21.8221, 39.3803) -> (22.1039, 39.6621)
  arc A2881 (22.031, 38.3394) -> (22.3329, 38.4375) centre (22.1819, 38.3884) ccw
  arc A2882 (22.0535, 38.1) -> (22.371, 38.1) centre (22.2123, 38.1) ccw
  arc A2883 (21.7194, 39.282) -> (21.5327, 39.0252) centre (21.626, 39.1536) ccw
  arc A2884 (21.4078, 39.3805) -> (21.5293, 39.0872) centre (21.4686, 39.2339) ccw
  line L938 (20.32, 38.1) -> (22.2123, 38.1)
  arc A2885 (22.3329, 37.7625) -> (22.031, 37.8606) centre (22.1819, 37.8116) ccw
  line L939 (22.2123, 38.1) -> (20.32, 38.1)
  arc A2886 (15.0857, 36.2682) -> (14.7923, 36.1467) centre (14.939, 36.2075) ccw
  arc A2887 (21.6896, 38.9112) -> (21.8762, 39.1681) centre (21.7829, 39.0397) ccw
  arc A2888 (22.3691, 37.9782) -> (22.0555, 38.0279) centre (22.2123, 38.0031) ccw
  line L940 (22.182, 37.8115) -> (22.2123, 38.003)
  line L941 (21.7829, 37.1604) -> (21.92, 37.2975)
  line L942 (22.2123, 38.197) -> (22.182, 38.3885)
  arc A2889 (20.4788, 38.1) -> (20.1613, 38.1) centre (20.3201, 38.1) ccw
  arc A2890 (22.0555, 38.1721) -> (22.3691, 38.2218) centre (22.2123, 38.197) ccw
  arc A2891 (25.5945, 39.5034) -> (25.5945, 39.8209) centre (25.5945, 39.6622) ccw
  line L943 (22.2123, 38.003) -> (22.2123, 38.1)
  line L944 (25.9539, 39.811) -> (26.5671, 40.4241)
  line L945 (22.2123, 38.1) -> (22.2123, 38.197)
  line L946 (21.6261, 39.1536) -> (21.4685, 39.2339)
  arc A2892 (25.5338, 39.8088) -> (25.6553, 39.5154) centre (25.5946, 39.6621) ccw
  arc A2893 (22.2123, 37.9412) -> (22.2123, 38.2587) centre (22.2123, 38.0999) ccw
  arc A2894 (22.0323, 37.1852) -> (21.8078, 37.4097) centre (21.92, 37.2975) ccw
  arc A2895 (20.1613, 38.1) -> (20.4788, 38.1) centre (20.3201, 38.1) ccw
  arc A2896 (22.2161, 39.5498) -> (21.9916, 39.7744) centre (22.1039, 39.6621) ccw
  line L947 (22.182, 38.3885) -> (22.122, 38.5729)
  line L948 (21.7829, 39.0396) -> (21.6261, 39.1536)
  line L949 (22.034, 37.4543) -> (22.122, 37.6271)
  line L950 (22.034, 38.7457) -> (21.92, 38.9025)
  arc A2897 (22.1039, 39.8209) -> (22.1039, 39.5034) centre (22.1039, 39.6622) ccw
  arc A2898 (21.8078, 38.7903) -> (22.0323, 39.0148) centre (21.92, 38.9026) ccw
  arc A2899 (21.8952, 39.1519) -> (21.6707, 38.9274) centre (21.783, 39.0396) ccw
  arc A2900 (22.2123, 37.9413) -> (22.2123, 38.2588) centre (22.2123, 38.1) ccw
  line L951 (21.92, 37.2975) -> (22.034, 37.4543)
  arc A2901 (22.0485, 38.9958) -> (21.7916, 38.8092) centre (21.92, 38.9025) ccw
  arc A2902 (21.7098, 39.4926) -> (21.9343, 39.2681) centre (21.822, 39.3803) ccw
  arc A2903 (22.1624, 37.361) -> (21.9056, 37.5477) centre (22.034, 37.4543) ccw
  arc A2904 (22.3388, 38.4133) -> (22.0252, 38.3636) centre (22.182, 38.3884) ccw
  arc A2905 (26.6793, 40.3118) -> (26.4548, 40.5364) centre (26.5671, 40.4241) ccw
  arc A2906 (21.6707, 37.2726) -> (21.8952, 37.0481) centre (21.783, 37.1603) ccw
  arc A2907 (22.371, 38.1) -> (22.0535, 38.1) centre (22.2123, 38.1) ccw
  line L952 (22.1039, 39.6621) -> (25.5945, 39.6621)
  line L953 (22.122, 37.6271) -> (22.182, 37.8115)
  arc A2908 (21.9056, 38.6523) -> (22.1624, 38.839) centre (22.034, 38.7457) ccw
  arc A2909 (21.8828, 39.2336) -> (21.7613, 39.527) centre (21.8221, 39.3803) ccw
  arc A2910 (21.9711, 37.6762) -> (22.273, 37.5781) centre (22.1221, 37.6272) ccw
  line L954 (25.5945, 39.6621) -> (25.9539, 39.811)
  arc A2911 (26.0147, 39.6643) -> (25.8932, 39.9576) centre (25.954, 39.8109) ccw
  arc A2912 (21.7916, 37.3908) -> (22.0485, 37.2042) centre (21.92, 37.2975) ccw
  line L955 (22.122, 38.5729) -> (22.034, 38.7457)
  line L956 (21.4685, 39.2339) -> (21.8221, 39.3803)
  arc A2913 (22.273, 38.6219) -> (21.9711, 38.5238) centre (22.1221, 38.5729) ccw
  arc A2914 (21.8926, 37.5264) -> (22.1755, 37.3823) centre (22.0341, 37.4544) ccw
  arc A2915 (20.32, 38.2587) -> (20.32, 37.9412) centre (20.32, 38.0999) ccw
  arc A2916 (22.2635, 37.555) -> (21.9806, 37.6992) centre (22.1221, 37.6271) ccw
  arc A2917 (22.0535, 38.003) -> (22.371, 38.003) centre (22.2123, 38.003) ccw
  arc A2918 (22.371, 38.197) -> (22.0535, 38.197) centre (22.2123, 38.197) ccw
  arc A2919 (22.1755, 38.8177) -> (21.8926, 38.6736) centre (22.0341, 38.7457) ccw
  arc A2920 (21.9806, 38.5008) -> (22.2635, 38.645) centre (22.1221, 38.5729) ccw
  line L957 (21.92, 38.9025) -> (21.7829, 39.0396)
  arc A2921 (37.4455, 43.2371) -> (37.4455, 43.5546) centre (37.4455, 43.3959) ccw
  arc A2922 (25.8417, 39.9232) -> (26.0662, 39.6987) centre (25.954, 39.811) ccw
  arc A2923 (38.1571, 41.2945) -> (38.4746, 41.2945) centre (38.3158, 41.2945) ccw
  arc A2924 (36.1023, 40.3118) -> (36.3268, 40.5364) centre (36.2145, 40.4241) ccw
  arc A2925 (27.1732, 40.5364) -> (27.3977, 40.3118) centre (27.2855, 40.4241) ccw
  arc A2926 (15.2717, 35.7874) -> (14.9542, 35.7874) centre (15.113, 35.7874) ccw
  arc A2927 (11.6574, 39.0842) -> (11.6574, 39.4017) centre (11.6574, 39.243) ccw
  arc A2928 (37.3332, 40.5364) -> (37.5577, 40.3118) centre (37.4455, 40.4241) ccw
  arc A2929 (36.2145, 43.5546) -> (36.2145, 43.2371) centre (36.2145, 43.3959) ccw
  arc A2930 (35.5029, 42.5255) -> (35.1854, 42.5255) centre (35.3441, 42.5255) ccw
  arc A2931 (12.2867, 38.6352) -> (12.5112, 38.8597) centre (12.399, 38.7475) ccw
  arc A2932 (4.3767, 40.6443) -> (4.1522, 40.4197) centre (4.2645, 40.532) ccw
  line L958 (15.113, 35.7874) -> (14.939, 36.2075)
  arc A2933 (14.7297, 36.6412) -> (14.5052, 36.4167) centre (14.6175, 36.529) ccw
  arc A2934 (14.5052, 36.4167) -> (14.7297, 36.6412) centre (14.6175, 36.529) ccw
  line L959 (37.4455, 40.4241) -> (38.3159, 41.2945)
  arc A2935 (15.5271, 34.9122) -> (15.2337, 34.7907) centre (15.3804, 34.8514) ccw
  arc A2936 (12.5112, 38.8597) -> (12.2867, 38.6352) centre (12.399, 38.7475) ccw
  line L960 (35.3441, 42.5255) -> (35.3441, 41.2945)
  arc A2937 (5.5534, 39.4017) -> (5.5534, 39.0842) centre (5.5534, 39.243) ccw
  arc A2938 (11.7181, 39.3897) -> (11.5966, 39.0963) centre (11.6573, 39.243) ccw
  line L961 (36.2145, 43.3959) -> (35.3441, 42.5255)
  arc A2939 (15.7924, 34.2399) -> (15.4749, 34.2399) centre (15.6337, 34.2399) ccw
  arc A2940 (35.2318, 42.6377) -> (35.4564, 42.4132) centre (35.3441, 42.5255) ccw
  line L962 (14.939, 36.2075) -> (14.6175, 36.529)
  line L963 (14.6175, 36.529) -> (12.399, 38.7475)
  line L964 (37.4455, 43.3959) -> (36.2145, 43.3959)
  line L965 (38.3159, 42.5255) -> (37.4455, 43.3959)
  arc A2941 (35.4564, 41.4068) -> (35.2318, 41.1823) centre (35.3441, 41.2946) ccw
  arc A2942 (28.2682, 41.1823) -> (28.0436, 41.4068) centre (28.1559, 41.2946) ccw
  line L966 (38.3159, 41.2945) -> (38.3159, 42.5255)
  arc A2943 (38.4282, 41.1823) -> (38.2036, 41.4068) centre (38.3159, 41.2945) ccw
  line L967 (12.399, 38.7475) -> (12.0775, 39.069)
  arc A2944 (14.8267, 36.0952) -> (15.0512, 36.3197) centre (14.939, 36.2075) ccw
  arc A2945 (27.2855, 40.2654) -> (27.2855, 40.5829) centre (27.2855, 40.4241) ccw
  line L968 (5.5534, 39.243) -> (4.2644, 40.532)
  arc A2946 (15.4749, 33.5781) -> (15.7924, 33.5781) centre (15.6337, 33.5781) ccw
  arc A2947 (15.487, 34.1792) -> (15.7804, 34.3007) centre (15.6337, 34.24) ccw
  line L969 (15.113, 35.1188) -> (15.113, 35.7874)